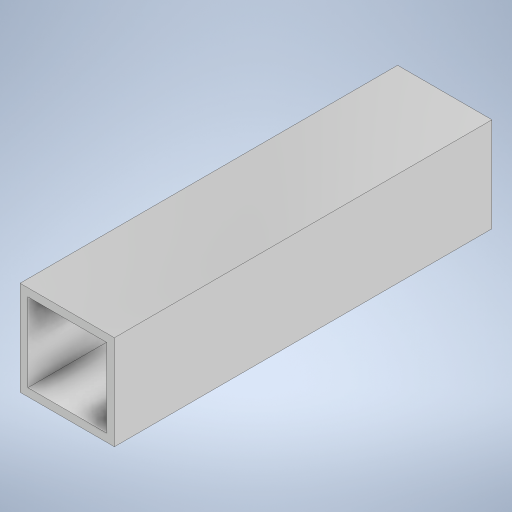
# Autodesk Inventor part: testRoboRescue_Chassis_Frame_lengthBar
Saved by Autodesk Inventor 2023 (Build 270158000, 158)
## iProperties
Created: 2022-03-14
Part Number: testRoboRescue_Chassis_Frame_lengthBar
Material: Aluminum 6061
Document SubType Name: Modeling
Designer: Nebil Oumer
Density: 2.7 g/cm^3
Appearance: Aluminum - Polished
Mass: 182.511 g
Surface Area: 434.677 cm^2
Volume: 67.5966 cm^3
Author: Nebil Oumer
Autodesk Inventor part; units mm, degrees
ref_plane "YZ Plane" through (0, 0, 0) normal (1, 0, 0) x (0, 1, 0)
ref_plane "XZ Plane" through (0, 0, 0) normal (0, 1, 0) x (-1, 0, 0)
ref_plane "XY Plane" through (0, 0, 0) normal (0, 0, 1) x (1, 0, 0)
sketch "Sketch1" plane through (0, 0, 0) normal (0, 0, 1) x (1, 0, 0)
  line L0 (0, 0) -> (38.1, 0)
  line L1 (38.1, 0) -> (38.1, 38.1)
  line L2 (38.1, 38.1) -> (0, 38.1)
  line L3 (0, 38.1) -> (0, 0)
  line L4 (34.925, 34.925) -> (34.925, 3.175)
  line L5 (34.925, 3.175) -> (3.175, 3.175)
  line L6 (3.175, 3.175) -> (3.175, 34.925)
  line L7 (3.175, 34.925) -> (34.925, 34.925)
  dimension "d0" = 38.1
  dimension "d1" = 38.1
  dimension "d2" = 3.175
  constraints: 16 end point, 4 parallel, 2 perpendicular, 1 horizontal, 3 other
  measures "d0" distance of L2.end L1.end
  measures "d1" distance of L0.end L1.end
  measures "d2" distance between parallel lines of L1 L4
extrude "Extrusion1" add sketch "Sketch1" along normal blind 152.4
equation "\"d0\" = d1"
body "Solid1"
